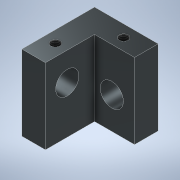
# Autodesk Inventor part: Laser Galvo Mount
Saved by Autodesk Inventor 2021 (Build 250183000, 183)
## iProperties
Created: 2021-04-06
Part Number: Laser Galvo Mount
Material: Generic
Document SubType Name: Modeling
Designer: Andrew
Density: 1 g/cm^3
Appearance: Smooth - Dark Forest Green
Author: Andrew
Autodesk Inventor part; units mm, degrees
ref_plane "YZ Plane" through (0, 0, 0) normal (1, 0, 0) x (0, 1, 0)
sketch "Body" plane through (0, 0, 0) normal (0, 1, 0) x (-1, 0, 0)
  line L0 (0, 0) -> (-35, 0)
  line L1 (-35, 0) -> (-35, 13)
  line L2 (-35, 13) -> (-13, 13)
  line L3 (-13, 13) -> (-13, 40)
  line L4 (-13, 40) -> (0, 40)
  line L5 (0, 40) -> (0, 0)
  circle A0 centre (-22.5, 6.5) radius 2.5
  circle A1 centre (-6.5, 28) radius 2.5
  point P0 (-35, 6.5)
  point P1 (-6.5, 40)
  dimension "d0" = 40
  dimension "d1" = 35
  dimension "d2" = 13
  dimension "d3" = 13
  dimension "d4" = 5
  dimension "d5" = 5
  dimension "d6" = 28
  dimension "d7" = 22.5
  constraints: 12 end point, 5 perpendicular, 2 centre point, 2 midpoint, 1 horizontal, 1 horizontal alignment, 1 vertical alignment
  measures "d0" distance of L4.end L0.start
  measures "d1" distance between parallel lines of L5 L1
  measures "d2" distance of L0.end L1.end
  measures "d3" distance of L3.end L4.end
  measures "d4" diameter of A0
  measures "d5" diameter of A1
  measures "d6" distance from line of A1.centre L0
  measures "d7" distance from line of A0.centre L5
extrude "Extrusion1" add sketch "Body" along normal blind 41.5 contours L0 L1 L2 L3 L4 L5 | A0 | A1
sketch "Lower Galvo Mount" plane through (35, 0, 0) normal (0, 0, -1) x (-1, 0, 0)
  circle A0 centre (12.5, 17.5) radius 6.375
  line L0 (0, 0) -> (35, 0) projected
  point P0 (12.5, 0)
  dimension "d10" = 17.5
  dimension "d11" = 12.75
  constraints: 1 centre point, 1 vertical alignment
  measures "d10" distance from line of L0 A0.centre
  measures "d11" diameter of A0
sketch "Upper Galvo Mount" plane through (0, 0, 0) normal (-1, 0, 0) x (0, 0, 1)
  circle A0 centre (28, 26) radius 6.375
  line L0 (0, 0) -> (40, 0) projected
  point P0 (28, 0)
  dimension "d12" = 12.75
  dimension "d13" = 26
  constraints: 1 centre point, 1 vertical alignment
  measures "d12" diameter of A0
  measures "d13" distance from line of L0 A0.centre
extrude "Extrusion2" cut sketch "Upper Galvo Mount" against normal through all
extrude "Extrusion3" cut sketch "Lower Galvo Mount" against normal through all
extrude "Extrusion4" cut sketch "Body" against normal up to surface from surface at 41.5 contours A0 round surface about axis through (22.5, 17.5, 0) along (0, 0, 1) radius 6.375 far side no
extrude "Extrusion5" cut sketch "Body" against normal up to surface from surface at 41.5 contours A1 round surface about axis through (0, 26, 28) along (1, 0, 0) radius 6.375 far side no
thread "Thread1" size "M5x0.8" class "6H" standard "ANSI Metric M Profile" full length
thread "Thread2" size "M5x0.8" class "6H" standard "ANSI Metric M Profile" full length
sketch "Sketch4" plane through (0, 0, 0) normal (0, -1, 0) x (1, 0, 0)
  circle A0 centre (5, 28) radius 1.75
  circle A1 centre (5, 15.5) radius 1.75
  circle A2 centre (29, 6.5) radius 1.75
  line L0 (35, 0) -> (0, 0) projected
  line L1 (0, 0) -> (0, 40) projected
  line L2 (35, 13) -> (35, 0) projected
  point P0 (35, 6.5)
  dimension "d26" = 28
  dimension "d27" = 15.5
  dimension "d28" = 29
  dimension "d29" = 3.5
  dimension "d30" = 3.5
  dimension "d31" = 3.5
  dimension "d32" = 5
  dimension "d35" = 35
  dimension "d36" = 40
  dimension "d37" = 13
  constraints: 3 centre point, 1 horizontal alignment, 1 midpoint, 1 vertical alignment
  measures "d26" distance from line of L0 A0.centre
  measures "d27" distance from line of L0 A1.centre
  measures "d28" distance from line of A2.centre L1
  measures "d29" diameter of A0
  measures "d30" diameter of A1
  measures "d31" diameter of A2
  measures "d32" distance from line of A0.centre L1
  measures "d35" distance of L0.start L0.end
  measures "d36" distance of L0.end L1.end
  measures "d37" distance of L2.start L0.start
extrude "Extrusion6" cut sketch "Sketch4" against normal blind 10
sketch "PCB Mount" plane through (0, 41.5, 0) normal (0, 1, 0) x (1, 0, 0)
  line L0 (0, 0) -> (120, 0)
  line L1 (120, 0) -> (120, -45)
  line L2 (120, -45) -> (0, -45)
  line L3 (0, -45) -> (0, 0)
  line L4 (0, -40) -> (13, -40) projected
  line L5 (0, -45) -> (-2.5, -45)
  line L6 (-2.5, -45) -> (-2.5, 2.5)
  line L7 (-2.5, 2.5) -> (120, 2.5)
  line L8 (120, 2.5) -> (120, 0)
  circle A0 centre (22.5, -6.5) radius 2.5 construction
  circle A1 centre (22.5, -6.5) radius 2.75
  dimension "d38" = 120
  dimension "d39" = 5
  dimension "d40" = 2.5
  dimension "d41" = 2.5
  dimension "d46" = 5.5
  constraints: 16 end point, 3 horizontal, 2 parallel, 2 perpendicular, 1 centre point, 1 coincident, 1 collinear
  measures "d38" distance of L0.start L0.end
  measures "d39" distance between parallel lines of L2 L4
  measures "d40" distance between parallel lines of L0 L7
  measures "d41" distance between parallel lines of L6 L3
  measures "d46" diameter of A1
extrude "Extrusion7" add sketch "PCB Mount" along normal blind 2.5 separate body
extrude "Extrusion8" add sketch "PCB Mount" against normal blind 5 contours L3 L5 L6 L7 L8 L0 bodies 2
chamfer "Chamfer1" distance 2.25 angle 45 1 edges at (19.75, 44, 6.5)
fillet "Fillet1" radius 5 1 edges at (120, 42.75, 45)
ref_plane "xaxisplane" through (22.5, 17.5, 13) normal (0.7660444, 0.6427876, 0) x (0, 0, -1)
ref_plane "yaxisplane" through (13, 26, 28) normal (0, 0.6427876, -0.7660444) x (-1, 0, 0)
ref_plane "projection plane" through (13, 26, 128) normal (0, 0, 1) x (-1, 0, 0)
ref_plane "Work Plane3" through (13, 26, 28) normal (0, 0, 1) x (-1, 0, 0)
sketch "Sketch6" plane through (13, 26, 28) normal (0, 0, 1) x (-1, 0, 0)
  line L0 (-9.5, 8.5) -> (-109.5, 8.5)
  line L1 (-9.5, 8.5) -> (-10.9988, 0)
  line L2 (29.2573, -37.6891) -> (-74.2166, 85.6263) construction
  line L3 (-134.5, 0) -> (40.5, 0) construction
  point P0 (13, 26)
  dimension "d55" = 100
  dimension "d60" = 80
  constraints: 4 end point, 1 coincident, 1 horizontal, 1 point on line
  measures "d55" distance of L0.start L0.end
  measures "d60" angle of L0 L1
ref_plane "Work Plane5" through (22.5, 17.5, 28) normal (0.9848078, -0.1736482, 0) x (0.1736482, 0.9848078, 0)
sketch "Sketch8" plane through (22.5, 17.5, 28) normal (0.9848078, -0.1736482, 0) x (0.1736482, 0.9848078, 0)
  line L0 (8.6311, 0) -> (26.2638, 100)
  line L1 (-38.4069, 100) -> (62.8677, 100) construction
  line L2 (-6.375, -15) -> (-6.375, -28) projected
  line L3 (0, 0) -> (8.6311, 0) projected
  line L4 (-6.375, -28) -> (-17.77, -28) projected
  line L5 (-17.77, -15) -> (-6.375, -15) projected
  line L6 (24.3702, -28) -> (6.375, -28) projected
  line L7 (-17.77, -28) -> (-17.77, -15) projected
  line L8 (24.3702, -15) -> (24.3702, -28) projected
  ellipse E0 centre (0, -21.5) end of major axis (-14.3969, -21.5) minor radius 2.5 (6.375, -23.7415) -> (6.375, -19.2585) ccw projected
  line L9 (6.375, -19.2585) -> (6.375, -15) projected
  line L10 (6.375, -15) -> (24.3702, -15) projected
  line L11 (6.375, -28) -> (6.375, -23.7415) projected
  point P0 (-21.1412, -28)
  dimension "d59" = 100
  constraints: 2 end point, 1 point on line, 1 other
  measures "d59" angle of L3 L0
equation "\"d59\" = 2 * y_axis_angle"
equation "\"d51\" = x_axis_angle"
equation "\"d52\" = y_axis_angle"
equation "\"y_axis_angle\" = 50deg"
equation "\"x_axis_angle\" = 50deg"
body "Solid1"
body "Solid2"
